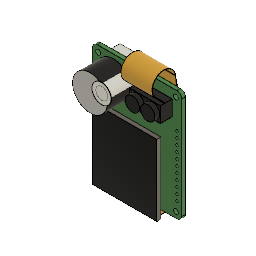
Sipeed MF1基板 v11 (Autodesk Fusion 360 design; units mm, degrees)
Autodesk Fusion 360 part; units mm, degrees
note: some values were not read from the file. Set by a fixed rule: which sketch regions a step uses.
sketch "スケッチ1" plane through (0, 0, 0) normal (0, 1, 0) x (1, 0, 0)
  line L0 (2, 0) -> (35.5, 0)
  line L1 (37.5, -2) -> (37.5, -44.7)
  line L2 (35.5, -46.7) -> (2, -46.7)
  line L3 (0, -44.7) -> (0, -2)
  arc A0 (0, -44.7) -> (2, -46.7) centre (2, -44.7) ccw
  arc A1 (35.5, -46.7) -> (37.5, -44.7) centre (35.5, -44.7) ccw
  arc A2 (37.5, -2) -> (35.5, 0) centre (35.5, -2) ccw
  arc A3 (2, 0) -> (0, -2) centre (2, -2) ccw
  circle A4 centre (2.45, -2.55) radius 1
  circle A5 centre (2.45, -44.15) radius 1
  circle A6 centre (35.05, -2.55) radius 1
  circle A7 centre (35.05, -44.15) radius 1
  line L4 (18.75, -46.7) -> (18.75, 0) construction
  line L5 (0, -23.35) -> (37.5, -23.35) construction
  circle A8 centre (2, -6.55) radius 1
  circle A9 centre (35.5, -6.55) radius 1
  circle A10 centre (2, -9.09) radius 1
  circle A11 centre (35.5, -9.09) radius 1
  circle A12 centre (2, -11.63) radius 1
  circle A13 centre (35.5, -11.63) radius 1
  circle A14 centre (2, -14.17) radius 1
  circle A15 centre (35.5, -14.17) radius 1
  circle A16 centre (2, -16.71) radius 1
  circle A17 centre (35.5, -16.71) radius 1
  circle A18 centre (2, -19.25) radius 1
  circle A19 centre (35.5, -19.25) radius 1
  circle A20 centre (2, -21.79) radius 1
  circle A21 centre (35.5, -21.79) radius 1
  circle A22 centre (2, -24.33) radius 1
  circle A23 centre (35.5, -24.33) radius 1
  circle A24 centre (2, -26.87) radius 1
  circle A25 centre (35.5, -26.87) radius 1
  circle A26 centre (2, -29.41) radius 1
  circle A27 centre (35.5, -29.41) radius 1
  circle A28 centre (2, -31.95) radius 1
  circle A29 centre (35.5, -31.95) radius 1
  circle A30 centre (2, -6.55) radius 0.5
  circle A31 centre (35.5, -6.55) radius 0.5
  circle A32 centre (2, -9.09) radius 0.5
  circle A33 centre (35.5, -9.09) radius 0.5
  circle A34 centre (2, -11.63) radius 0.5
  circle A35 centre (35.5, -11.63) radius 0.5
  circle A36 centre (2, -14.17) radius 0.5
  circle A37 centre (35.5, -14.17) radius 0.5
  circle A38 centre (2, -16.71) radius 0.5
  circle A39 centre (35.5, -16.71) radius 0.5
  circle A40 centre (2, -19.25) radius 0.5
  circle A41 centre (35.5, -19.25) radius 0.5
  circle A42 centre (2, -21.79) radius 0.5
  circle A43 centre (35.5, -21.79) radius 0.5
  circle A44 centre (2, -24.33) radius 0.5
  circle A45 centre (35.5, -24.33) radius 0.5
  circle A46 centre (2, -26.87) radius 0.5
  circle A47 centre (35.5, -26.87) radius 0.5
  circle A48 centre (2, -29.41) radius 0.5
  circle A49 centre (35.5, -29.41) radius 0.5
  circle A50 centre (2, -31.95) radius 0.5
  circle A51 centre (35.5, -31.95) radius 0.5
  point P0 (37.5, 0)
  point P1 (0, -46.7)
  dimension "d1" = 37.5
  dimension "d2" = 46.7
  dimension "d3" = 2
  dimension "d4" = 2
  dimension "d5" = 2
  dimension "d6" = 41.6
  dimension "d9" = 32.6
  dimension "d10" = 0
  dimension "d11" = 32.6
  dimension "d12" = 32.6
  dimension "d13" = 16.3
  dimension "d14" = 20.8
  dimension "d34" = 2
  dimension "d35" = 2
  dimension "d36" = 4
  dimension "d39" = 33.5
  dimension "d40" = -25.4
  dimension "d41" = 1
  dimension "d44" = 33.5
  dimension "d45" = -25.4
  constraint horizontal L0
  constraint vertical L1
  constraint horizontal L2
  constraint vertical L3
  constraint coincident P1 L2
  constraint coincident P1 L3
  constraint tangent L2 A0
  constraint tangent L3 A0
  constraint tangent L1 A1
  constraint tangent L2 A1
  constraint equal A0 A1
  constraint coincident P0 L0
  constraint coincident P0 L1
  constraint tangent L0 A2
  constraint tangent L1 A2
  constraint equal A0 A2
  constraint coincident origin L0
  constraint coincident origin L3
  constraint tangent L0 A3
  constraint tangent L3 A3
  constraint equal A0 A3
  constraint midpoint L2 L4.start
  constraint midpoint L0 L4.end
  constraint midpoint L3 L5.start
  constraint midpoint L1 L5.end
  constraint concentric A8 A30
  measures "d1" distance of origin P0
  measures "d2" distance of origin P1
  measures "d3" radius of A0
  measures "d4" diameter of A4
  measures "d5" diameter of A5
  measures "d6" distance of A4.centre A5.centre
  measures "d11" distance of A4.centre A6.centre
  measures "d12" distance of A5.centre A7.centre
  measures "d13" distance of A6.centre L4
  measures "d14" distance of A6.centre L5
  measures "d34" diameter of A8
  measures "d35" distance of L3 A8.centre
  measures "d36" vertical distance of A4.centre A8.centre
  measures "d41" diameter of A30
extrude "押し出し1" add sketch "スケッチ1" along normal blind 1.6 contours L0 L1 L2 L3 A0 A1 A2 A3 | A8 | A9 | A10 | A11 | A12 | A13 | A14 | A15 | A16 | A17 | A18 | A19 | A20 | A21 | A22 | A23 | A24 | A25 | A26 | A27 | A28 | A29 | A30 | A31 | A32 | A33 | A34 | A35 | A36 | A37 | A38 | A39 | A40 | A41 | A42 | A43 | A44 | A45 | A46 | A47 | A48 | A49 | A50 | A51 makes body 1
sketch "スケッチ2" plane through (0, 0, 0) normal (0, -1, 0) x (1, 0, 0)
  circle A0 centre (2.45, 44.15) radius 1
  circle A1 centre (35.05, 44.15) radius 1
  circle A2 centre (35.05, 2.55) radius 1
  circle A3 centre (2.45, 2.55) radius 1
  arc A4 (35.5, 0) -> (37.5, 2) centre (35.5, 2) ccw
  line L0 (37.5, 2) -> (37.5, 44.7)
  arc A5 (37.5, 44.7) -> (35.5, 46.7) centre (35.5, 44.7) ccw
  line L1 (35.5, 46.7) -> (2, 46.7)
  arc A6 (2, 46.7) -> (0, 44.7) centre (2, 44.7) ccw
  line L2 (0, 44.7) -> (0, 2)
  arc A7 (0, 2) -> (2, 0) centre (2, 2) ccw
  line L3 (2, 0) -> (35.5, 0)
  circle A8 centre (8.95, 37.65) radius 7.325
  line L4 (5.25, 0) -> (32.25, 0)
  line L5 (32.25, 0) -> (32.25, 30)
  line L6 (32.25, 30) -> (5.25, 30)
  line L7 (5.25, 30) -> (5.25, 0)
  line L8 (18.75, 46.7) -> (18.75, 0)
  line L9 (20.5, 42.7) -> (33.5, 42.7)
  line L10 (33.5, 42.7) -> (33.5, 36.2)
  line L11 (33.5, 36.2) -> (20.5, 36.2)
  line L12 (20.5, 36.2) -> (20.5, 42.7)
  line L13 (37.5, 2) -> (37.5, 44.7)
  line L14 (35.5, 46.7) -> (2, 46.7)
  line L15 (27, 36.2) -> (27, 42.7)
  line L16 (27, 36.2) -> (33.5, 36.2)
  line L17 (33.5, 36.2) -> (33.5, 42.7)
  line L18 (33.5, 42.7) -> (27, 42.7)
  line L19 (27, 42.7) -> (27, 36.2)
  line L20 (27, 42.7) -> (20.5, 42.7)
  line L21 (20.5, 42.7) -> (20.5, 36.2)
  line L22 (20.5, 36.2) -> (27, 36.2)
  line L23 (27, 36.2) -> (27, 42.7)
  circle A9 centre (23.75, 39.45) radius 3
  circle A10 centre (30.25, 39.45) radius 3
  circle A11 centre (18, 44) radius 2.5
  point P0 (18.75, 30)
  dimension "d17" = 14.65
  dimension "d18" = 6.5
  dimension "d19" = 6.5
  dimension "d22" = 27
  dimension "d23" = 30
  dimension "d48" = 13
  dimension "d49" = 6.5
  dimension "d50" = 4
  dimension "d51" = 4
  dimension "d52" = 6
  dimension "d53" = 6
  dimension "d72" = 5
  constraint horizontal L4
  constraint vertical L5
  constraint horizontal L6
  constraint vertical L7
  constraint coincident L3 L4.start
  constraint midpoint L6 P0
  constraint coincident P0 L8
  constraint horizontal L9
  constraint vertical L10
  constraint horizontal L11
  constraint vertical L12
  constraint midpoint L11 L15.start
  constraint midpoint L9 L15.end
  constraint horizontal L16
  constraint vertical L17
  constraint horizontal L18
  constraint vertical L19
  constraint horizontal L20
  constraint vertical L21
  constraint horizontal L22
  constraint vertical L23
  measures "d17" diameter of A8
  measures "d18" horizontal distance of A0.centre A8.centre
  measures "d19" vertical distance of A0.centre A8.centre
  measures "d22" distance of L5.end L6.end
  measures "d23" distance of L4.end L5.end
  measures "d48" distance of L10.end L11.end
  measures "d49" distance of L9.end L10.end
  measures "d50" distance of L10 L13
  measures "d51" distance of L9 L14
  measures "d52" diameter of A9
  measures "d53" diameter of A10
  measures "d72" diameter of A11
extrude "押し出し3" add sketch "スケッチ2" along normal blind 1.7 from surface at 3.5 separate body contours L3 L4 L5 L6 L8 | L3 L4 L6 L7 L8 makes body 2
extrude "押し出し2" add sketch "スケッチ2" along normal blind 10 separate body contours A8 makes body 3
sketch "スケッチ3" plane through (0, 1.6, 0) normal (0, 1, 0) x (-1, 0, 0)
  circle A0 centre (-2.45, 44.15) radius 1
  circle A1 centre (-35.05, 44.15) radius 1
  circle A2 centre (-35.05, 2.55) radius 1
  circle A3 centre (-2.45, 2.55) radius 1
  arc A4 (-37.5, 2) -> (-35.5, 0) centre (-35.5, 2) ccw
  line L0 (-35.5, 0) -> (-2, 0)
  arc A5 (-2, 0) -> (0, 2) centre (-2, 2) ccw
  line L1 (0, 2) -> (0, 44.7)
  arc A6 (0, 44.7) -> (-2, 46.7) centre (-2, 44.7) ccw
  line L2 (-2, 46.7) -> (-35.5, 46.7)
  arc A7 (-35.5, 46.7) -> (-37.5, 44.7) centre (-35.5, 44.7) ccw
  line L3 (-37.5, 44.7) -> (-37.5, 2)
  line L4 (-4, 0) -> (-13, 0)
  line L5 (-13, 0) -> (-13, 8)
  line L6 (-13, 8) -> (-4, 8)
  line L7 (-4, 8) -> (-4, 0)
  line L8 (0, 44.7) -> (0, 2)
  line L9 (-13, 45.3) -> (-5, 45.3)
  line L10 (-5, 45.3) -> (-5, 41.3)
  line L11 (-5, 41.3) -> (-13, 41.3)
  line L12 (-13, 41.3) -> (-13, 45.3)
  line L13 (-35.5, 46.7) -> (-2, 46.7)
  point P0 (-8.5, 8)
  dimension "d27" = 9
  dimension "d28" = 8
  dimension "d29" = 8.5
  dimension "d66" = 8
  dimension "d67" = 4
  dimension "d68" = 1.4
  dimension "d69" = 5
  constraint horizontal L4
  constraint vertical L5
  constraint horizontal L6
  constraint vertical L7
  constraint coincident L0 L4.start
  constraint midpoint L6 P0
  constraint horizontal L9
  constraint vertical L10
  constraint horizontal L11
  constraint vertical L12
  measures "d27" distance of L5.end L6.end
  measures "d28" distance of L4.end L5.end
  measures "d29" distance of P0 L8
  measures "d66" distance of L9.start L9.end
  measures "d67" distance of L9.start L11.end
  measures "d68" distance of L9 L13
  measures "d69" distance of L8 L10
extrude "押し出し4" add sketch "スケッチ3" along normal blind 3 separate body contours L0 L4 L5 L6 L7 makes body 4
fillet "フィレット1" radius 1 1 edges at (13, 4.6, 4) on bodies 4
fillet "フィレット2" radius 1 3 edges at (4, 1.6, 4) (4, 4.6, 4) (13, 1.6, 4) on bodies 4
extrude "押し出し5" cut sketch "スケッチ1" along normal blind 11 contours A30 | A31 | A32 | A33 | A34 | A35 | A36 | A37 | A38 | A39 | A40 | A41 | A42 | A43 | A44 | A45 | A46 | A47 | A48 | A49 | A50 | A51 bodies 1
extrude "押し出し6" add sketch "スケッチ2" along normal blind 5 separate body contours L9 L11 L12 L15 L19 L20 L21 L22 L23 | L9 L10 L11 L15 L16 L17 L18 L19 L23 makes body 5
extrude "押し出し7" add sketch "スケッチ2" along normal blind 7 contours A9 | A10 bodies 5
sketch "スケッチ4" plane through (32.25, 0, 0) normal (1, 0, 0) x (0, 1, 0)
  line L0 (-3.5, 0) -> (-3.5, 30)
  line L1 (-3.5, 30) -> (-5.2, 30)
  line L2 (-5.2, 30) -> (-5.2, 0)
  line L3 (-5.2, 0) -> (-3.5, 0)
  line L4 (1.8235, -1.179) -> (-1.833, -1.6918)
  line L5 (-1.8283, -1.4901) -> (1.7674, -0.9859)
  line L6 (-3.5, 0) -> (-3.7, 0)
  line L7 (2.6, 0) -> (2.8, 0)
  arc A0 (1.7103, -0.9939) -> (2.6, 0) centre (1.6, 0) ccw
  arc A1 (1.7094, -1.195) -> (2.8, 0) centre (1.6, 0) ccw
  arc A2 (-3.7, 0) -> (-1.6952, -1.6725) centre (-2, 0) ccw
  arc A3 (-3.5, 0) -> (-1.7552, -1.4799) centre (-2, 0) ccw
  constraint tangent L0 A3
  constraint coincident L4.start A1
  constraint coincident L4.end A2
  constraint coincident L5.start A3
  constraint parallel L4 L5
  constraint coincident L0.start L3.end
  constraint coincident L3 L6.end
  constraint horizontal L7
  constraint coincident L5.end A0
  constraint coincident L5 A0.start
  constraint coincident L4 A1.start
  constraint concentric A2 A3
  constraint coincident L5 A3.end
  constraint coincident L4 A2.end
extrude "押し出し8" add sketch "スケッチ4" against normal blind 14 from surface at -3 separate body contours L3 L4 L5 L6 L7 A0 A1 A2 A3 makes body 6
sketch "スケッチ5" plane through (33.5, 0, 0) normal (1, 0, 0) x (0, 1, 0)
  line L0 (0, 36.2) -> (0, 42.7)
  line L1 (0, 42.7) -> (-5, 42.7)
  line L2 (-5, 42.7) -> (-5, 36.2)
  line L3 (-5, 36.2) -> (0, 36.2)
  line L4 (-7.2564, 46.7) -> (-3.2651, 42.7)
  line L5 (-6.8692, 46.5812) -> (-2.9966, 42.7)
  line L6 (-3.2651, 42.7) -> (-2.9966, 42.7)
  line L7 (1.196, 50.9937) -> (2, 46)
  line L8 (2, 46) -> (2.3716, 46)
  line L9 (2.3716, 46) -> (1.4484, 50.7164)
  arc A0 (1.4484, 50.7164) -> (-6.8082, 46.2509) centre (-3.5, 50) ccw
  arc A1 (1.2706, 50.5304) -> (-6.8692, 46.5812) centre (-3.5, 50) ccw
  constraint coincident L4.start A0
  constraint coincident L1 L4.end
  constraint coincident L1 L5.end
  constraint parallel L4 L5
  constraint coincident L7.start A1
  constraint horizontal L8
  constraint coincident L7 A1.start
  constraint coincident L4 A0.end
extrude "押し出し9" add sketch "スケッチ5" against normal blind 13 separate body contours L1 L4 L5 L6 L7 L8 L9 A0 A1 makes body 7
extrude "押し出し10" add sketch "スケッチ3" along normal blind 5 separate body contours L9 L10 L11 L12 makes body 8
extrude "押し出し11" add sketch "スケッチ2" along normal blind 0.2 separate body contours L8 A11 | L8 A11 makes body 9
ref_plane "作業平面1" through (18, -14.2, 44) normal (0, -1, 0) x (1, 0, 0)
sketch "スケッチ6" plane through (18, -14.2, 44) normal (0, -1, 0) x (1, 0, 0)
  circle A0 centre (0, 0) radius 4
  dimension "d76" = 8
  constraint coincident A0.centre origin
  measures "d76" diameter of A0
extrude "押し出し12" add sketch "スケッチ6" against normal blind 0.2 separate body makes body 10
extrude "押し出し13" add 1 faces at (17.6897, -0.2, 43.238) along direction (0, -1, 0) blind 14 on bodies 9 bodies 9 10
named bodies: "基板", "ライト", "液晶", "USB-C", "カメラ", "フレキ1", "フレキ2", "背面コネクタ", "スプリングスイッチ"
